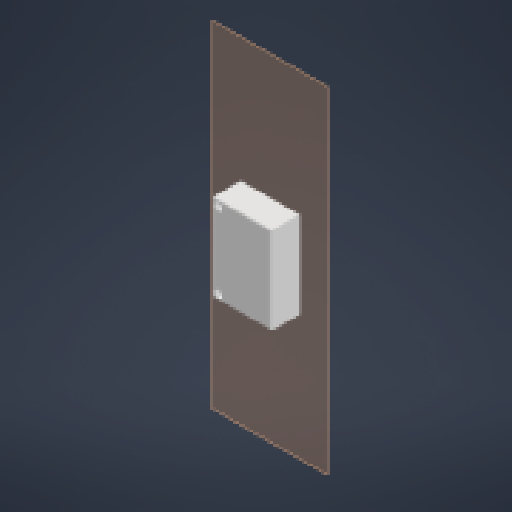
# Autodesk Inventor part: optoNCDT_mount
Saved by Autodesk Inventor 2027.1 (Build 311270010, 270A)
## iProperties
Created: 2026-09-14
Part Number: optoNCDT_mount
Material: Generic
Document SubType Name: Modeling
Designer: Jacob Parker
Density: 1 g/cm^3
Appearance: Default
Author: Jacob Parker
Autodesk Inventor part; units mm, degrees
ref_plane "YZ Plane" through (0, 0, 0) normal (1, 0, 0) x (0, 1, 0)
ref_plane "XZ Plane" through (0, 0, 0) normal (0, 1, 0) x (-1, 0, 0)
ref_plane "XY Plane" through (0, 0, 0) normal (0, 0, 1) x (1, 0, 0)
ref_plane "Work Plane1" through (0, 0, 0) normal (0, 0, 1) x (1, 0, 0)
sketch "SKbase" plane through (0, 0, 0) normal (0, 0, 1) x (1, 0, 0)
  line L0 (15.5, 23) -> (-15.5, 23)
  line L1 (-15.5, 23) -> (-15.5, -23)
  line L2 (-15.5, -23) -> (15.5, -23)
  line L3 (15.5, -23) -> (15.5, 23)
  point P0 (0, 0)
  point P1 (15.5, 0)
  point P2 (0, -23)
  dimension "d0" = 31
  dimension "d1" = 46
  dimension "d2" = 0
  dimension "d3" = 0
  constraints: 8 end point, 2 midpoint, 2 parallel, 1 horizontal, 1 perpendicular
  measures "d0" distance of L2.end L1.end
  measures "d1" distance of L2.end L0.start
  measures "d2" vertical distance of point (0, 0) point (15.5, 0)
  measures "d3" horizontal distance of point (0, 0) point (0, -23)
extrude "EXbase" add sketch "SKbase" along normal blind 15
sketch "Sketch2" plane through (0, 0, 15) normal (0, 0, 1) x (1, 0, 0)
  line L0 (-12.4313, 20) -> (-12.4313, 23)
  line L1 (15.5, 23) -> (-15.5, 23) projected
  line L2 (-12.4313, -20) -> (-12.4313, -23)
  line L3 (-15.5, -23) -> (15.5, -23) projected
  point P0 (0, 0)
  dimension "d6" = 40
  constraints: 4 end point, 2 point on line, 2 vertical, 1 collinear
  measures "d6" distance of L0.start L2.start
hole "Hole1" at (-12.4313, -20, 15) at (-12.4313, 20, 15) direction (0, 0, -1) diameter 4 end through all
fillet "Fillet1" radius 1 4 edges at (15.5, 0, 15) (0, 23, 15) (-15.5, 0, 15) (0, -23, 15)
sketch "Sketch3" plane through (0, 0, 0) normal (0, 0, -1) x (-1, 0, 0)
  circle A0 centre (12.4313, 20) radius 2 projected
  circle A1 centre (12.4313, -20) radius 2 projected
  point P0 (0, 0)
hole "Hole2" at (-12.4313, 20, 0) at (-12.4313, -20, 0) direction (0, 0, 1) diameter 6 depth 12
body "Solid1"
